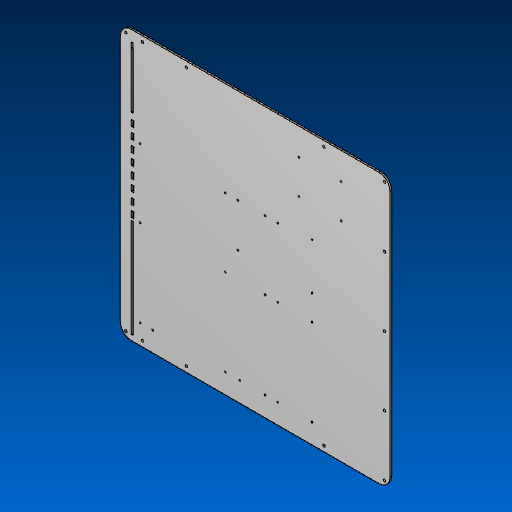
# Autodesk Inventor part: right_panel
Saved by Autodesk Inventor 2018 (Build 220112000, 112)
## iProperties
Created: 2019-10-14
Part Number: right_panel
Material: アルミニウム 6061
Document SubType Name: Modeling
Designer: gisen
Density: 2.7 g/cm^3
Appearance: アルミニウム - フラット
Author: gisen
Autodesk Inventor part; units mm, degrees
ref_plane "YZ Plane" through (0, 0, 0) normal (1, 0, 0) x (0, 1, 0)
ref_plane "XZ Plane" through (0, 0, 0) normal (0, 1, 0) x (-1, 0, 0)
ref_plane "XY Plane" through (0, 0, 0) normal (0, 0, 1) x (1, 0, 0)
sketch "スケッチ1" plane through (0, 0, 0) normal (0, 0, 1) x (1, 0, 0)
  line L0 (-225, -245) -> (225, -245)
  line L1 (245, -225) -> (245, 225)
  line L2 (225, 245) -> (-225, 245)
  line L3 (-245, 225) -> (-245, -225)
  line L4 (-245, -245) -> (245, 245) construction
  line L5 (245, -245) -> (-245, 245) construction
  circle A0 centre (-235, 235) radius 2.25
  circle A1 centre (235, 235) radius 2.25
  circle A2 centre (-235, -235) radius 2.25
  circle A3 centre (235, -235) radius 2.25
  arc A4 (-225, 245) -> (-245, 225) centre (-225, 225) ccw
  arc A5 (245, 225) -> (225, 245) centre (225, 225) ccw
  arc A6 (225, -245) -> (245, -225) centre (225, -225) ccw
  arc A7 (-245, -225) -> (-225, -245) centre (-225, -225) ccw
  point P0 (0, 0)
  dimension "d0" = 490
  dimension "d1" = 490
  dimension "d2" = 4.5
  dimension "d3" = 10
  dimension "d4" = 10
  dimension "d5" = 10
  dimension "d6" = 10
  dimension "d7" = 10
  dimension "d8" = 10
  dimension "d9" = 10
  dimension "d10" = 10
  dimension "d11" = 20
  constraints: 12 end point, 8 centre point, 8 point on circle, 8 point on line, 8 tangent, 6 equal radius, 2 midpoint, 2 parallel, 1 horizontal, 1 perpendicular
  measures "d0" distance of L5.end L4.end
  measures "d1" distance of L4.end L5.start
  measures "d2" diameter of A0
  measures "d3" distance from line of A0.centre L2
  measures "d4" distance from line of L3 A0.centre
  measures "d5" distance from line of A1.centre L2
  measures "d6" distance from line of L1 A1.centre
  measures "d7" distance from line of L1 A3.centre
  measures "d8" distance from line of L0 A3.centre
  measures "d9" distance from line of L0 A2.centre
  measures "d10" distance from line of L3 A2.centre
  measures "d11" radius of A4
extrude "押し出し1" add sketch "スケッチ1" along normal blind 3
sketch "スケッチ2" plane through (0, 0, 3) normal (0, 0, 1) x (1, 0, 0)
  circle A0 centre (18.0923, 72.9265) radius 1.6
  circle A1 centre (-54.2977, 72.9265) radius 1.6
  circle A2 centre (-209.2377, 72.9265) radius 1.6
  circle A3 centre (-209.2377, -51.5335) radius 1.6
  circle A4 centre (-186.3777, -209.0135) radius 1.6
  circle A5 centre (-54.2977, -209.0135) radius 1.6
  circle A6 centre (18.0923, -209.0135) radius 1.6
  circle A7 centre (18.0923, -51.5335) radius 1.6
  circle A8 centre (-54.2977, -51.5335) radius 1.6
  circle A9 centre (18.092, -209.014) radius 2.25 projected
  circle A10 centre (-186.378, -209.014) radius 2.25 projected
  circle A11 centre (18.092, -51.534) radius 2.25 projected
  circle A12 centre (18.092, 72.926) radius 2.25 projected
  circle A13 centre (-54.298, -209.014) radius 2.25 projected
  circle A14 centre (-54.298, -51.534) radius 2.25 projected
  circle A15 centre (-54.298, 72.926) radius 2.25 projected
  circle A16 centre (-209.238, -51.534) radius 2.25 projected
  circle A17 centre (-209.238, 72.926) radius 2.25 projected
  point P0 (0, 0)
  dimension "d14" = 3.2
  constraints: 9 centre point, 8 equal radius
  measures "d14" diameter of A0
extrude "押し出し2" cut sketch "スケッチ2" against normal blind 3 contours A0 | A1 | A2 | A3 | A4 | A5 | A6 | A7 | A8
sketch "スケッチ4" plane through (0, 0, 3) normal (0, 0, 1) x (1, 0, 0)
  line L0 (-225, -225) -> (-222, -225) projected
  line L1 (-225, -50.8937) -> (-225, -40.6067) projected
  line L2 (-225, -50.8937) -> (-222, -50.8937) projected
  line L3 (-222, -40.6067) -> (-222, -50.8937) projected
  line L4 (-225, -40.6067) -> (-222, -40.6067) projected
  line L5 (-225, -30.5483) -> (-225, -20.2613) projected
  line L6 (-225, -30.5483) -> (-222, -30.5483) projected
  line L7 (-222, -20.2613) -> (-222, -30.5483) projected
  line L8 (-225, -20.2613) -> (-222, -20.2613) projected
  line L9 (-225, -9.8937) -> (-225, 0.3933) projected
  line L10 (-225, -9.8937) -> (-222, -9.8937) projected
  line L11 (-222, 0.3933) -> (-222, -9.8937) projected
  line L12 (-225, 0.3933) -> (-222, 0.3933) projected
  line L13 (-225, 10.4517) -> (-225, 20.7387) projected
  line L14 (-225, 10.4517) -> (-222, 10.4517) projected
  line L15 (-222, 20.7387) -> (-222, 10.4517) projected
  line L16 (-225, 20.7387) -> (-222, 20.7387) projected
  line L17 (-225, 31.1063) -> (-225, 41.3933) projected
  line L18 (-225, 31.1063) -> (-222, 31.1063) projected
  line L19 (-222, 41.3933) -> (-222, 31.1063) projected
  line L20 (-225, 41.3933) -> (-222, 41.3933) projected
  line L21 (-225, 51.4517) -> (-225, 61.7387) projected
  line L22 (-225, 51.4517) -> (-222, 51.4517) projected
  line L23 (-222, 61.7387) -> (-222, 51.4517) projected
  line L24 (-225, 61.7387) -> (-222, 61.7387) projected
  line L25 (-225, 72.1063) -> (-225, 82.3933) projected
  line L26 (-225, 72.1063) -> (-222, 72.1063) projected
  line L27 (-222, 82.3933) -> (-222, 72.1063) projected
  line L28 (-225, 82.3933) -> (-222, 82.3933) projected
  line L29 (-225, 92.4517) -> (-225, 102.7387) projected
  line L30 (-225, 92.4517) -> (-222, 92.4517) projected
  line L31 (-222, 102.7387) -> (-222, 92.4517) projected
  line L32 (-225, 102.7387) -> (-222, 102.7387) projected
  line L33 (-225, 225) -> (-225, 132.6) projected
  line L34 (-225, 132.6) -> (-222, 132.6) projected
  line L35 (-222, 225) -> (-222, 132.6) projected
  line L36 (-225, 225) -> (-222, 225) projected
  line L37 (-222, 102.7387) -> (-221, 102.7387)
  line L38 (-221, 102.7387) -> (-221, 92.4517)
  line L39 (-221, 92.4517) -> (-222, 92.4517)
  line L40 (-222, 82.3933) -> (-221, 82.3933)
  line L41 (-221, 82.3933) -> (-221, 72.1063)
  line L42 (-221, 72.1063) -> (-222, 72.1063)
  line L43 (-222, 61.7387) -> (-221, 61.7387)
  line L44 (-221, 61.7387) -> (-221, 51.4517)
  line L45 (-221, 51.4517) -> (-222, 51.4517)
  line L46 (-222, 41.3933) -> (-221, 41.3933)
  line L47 (-221, 41.3933) -> (-221, 31.1063)
  line L48 (-221, 31.1063) -> (-222, 31.1063)
  line L49 (-222, 20.7387) -> (-221, 20.7387)
  line L50 (-221, 20.7387) -> (-221, 10.4517)
  line L51 (-221, 10.4517) -> (-222, 10.4517)
  line L52 (-222, 0.3933) -> (-221, 0.3933)
  line L53 (-221, 0.3933) -> (-221, -9.8937)
  line L54 (-221, -9.8937) -> (-222, -9.8937)
  line L55 (-222, -20.2613) -> (-221, -20.2613)
  line L56 (-221, -20.2613) -> (-221, -30.5483)
  line L57 (-221, -30.5483) -> (-222, -30.5483)
  line L58 (-222, -40.6067) -> (-221, -40.6067)
  line L59 (-221, -40.6067) -> (-221, -50.8937)
  line L60 (-221, -50.8937) -> (-222, -50.8937)
  line L61 (-225, -225) -> (-225, -56.064) projected
  line L62 (-222, -56.064) -> (-222, -225) projected
  line L63 (-225, -56.064) -> (-222, -56.064) projected
  point P0 (0, 0)
  point P1 (-225, -58.3552)
  point P2 (-222, -58.3552)
  point P3 (-225, -120.4005)
  point P4 (-222, -120.4005)
  dimension "d17" = 1
  constraints: 48 end point, 15 perpendicular, 8 horizontal, 7 parallel, 1 collinear, 2 other
  measures "d17" distance of L31.start L37.end
extrude "押し出し3" cut sketch "スケッチ4" against normal blind 3
sketch "スケッチ5" plane through (0, 0, 3) normal (0, 0, 1) x (1, 0, 0)
  circle A0 centre (-235, 235) radius 2.25 construction
  circle A1 centre (-235, -235) radius 2.25 construction
  circle A2 centre (-205, -235) radius 2.25
  line L0 (-225, -245) -> (225, -245) projected
  circle A3 centre (-205, 235) radius 2.25
  line L1 (225, 245) -> (-225, 245) projected
  point P0 (0, 0)
  dimension "d20" = 30
  dimension "d21" = 10
  dimension "d22" = 30
  dimension "d23" = 10
  constraints: 2 centre point, 2 equal radius
  measures "d20" distance of A1.centre A2.centre
  measures "d21" distance from line of L0 A2.centre
  measures "d22" distance of A0.centre A3.centre
  measures "d23" distance from line of L1 A3.centre
extrude "押し出し4" cut sketch "スケッチ5" against normal blind 3
sketch "スケッチ6" plane through (0, 0, 3) normal (0, 0, 1) x (1, 0, 0)
  circle A0 centre (-205, -235) radius 2.25 construction
  circle A1 centre (-205, 235) radius 2.25 construction
  circle A2 centre (18.0923, -51.5335) radius 1.6 construction
  circle A3 centre (-54.2977, -209.0135) radius 1.6 construction
  circle A4 centre (-209.2377, -51.5335) radius 1.6 construction
  circle A5 centre (-54.2977, 72.9265) radius 1.6 construction
  circle A6 centre (18.0923, 72.9265) radius 1.6 construction
  circle A7 centre (-209.2377, 72.9265) radius 1.6 construction
  circle A8 centre (-186.3777, -209.0135) radius 1.6 construction
  circle A9 centre (18.0923, -209.0135) radius 1.6 construction
  circle A10 centre (-54.2977, -51.5335) radius 1.6 construction
  circle A11 centre (235, -235) radius 2.25 construction
  circle A12 centre (-235, -235) radius 2.25 construction
  circle A13 centre (235, 235) radius 2.25 construction
  circle A14 centre (-235, 235) radius 2.25 construction
  line L0 (225, 245) -> (-225, 245) construction
  arc A15 (-225, 245) -> (-245, 225) centre (-225, 225) ccw construction
  line L1 (-245, 225) -> (-245, -225) construction
  arc A16 (-245, -225) -> (-225, -245) centre (-225, -225) ccw construction
  line L2 (-225, -245) -> (225, -245) construction
  arc A17 (225, -245) -> (245, -225) centre (225, -225) ccw construction
  line L3 (245, -225) -> (245, 225) construction
  arc A18 (245, 225) -> (225, 245) centre (225, 225) ccw construction
  line L4 (-221.75, 114.35) -> (-225.25, 114.35)
  line L5 (-225.25, 114.35) -> (-225.25, 215.25)
  line L6 (-225.25, 215.25) -> (-221.75, 215.25)
  line L7 (-221.75, 215.25) -> (-221.75, 114.35)
  line L8 (-220.75, 102.9892) -> (-220.75, 92.2022)
  line L9 (-220.75, 92.2022) -> (-225.25, 92.2022)
  line L10 (-225.25, 92.2022) -> (-225.25, 102.9892)
  line L11 (-225.25, 102.9892) -> (-220.75, 102.9892)
  line L12 (-220.75, 82.6438) -> (-220.75, 71.8568)
  line L13 (-220.75, 71.8568) -> (-225.25, 71.8568)
  line L14 (-225.25, 71.8568) -> (-225.25, 82.6438)
  line L15 (-225.25, 82.6438) -> (-220.75, 82.6438)
  line L16 (-220.75, 61.9892) -> (-220.75, 51.2022)
  line L17 (-220.75, 51.2022) -> (-225.25, 51.2022)
  line L18 (-225.25, 51.2022) -> (-225.25, 61.9892)
  line L19 (-225.25, 61.9892) -> (-220.75, 61.9892)
  line L20 (-220.75, 41.6438) -> (-220.75, 30.8568)
  line L21 (-220.75, 30.8568) -> (-225.25, 30.8568)
  line L22 (-225.25, 30.8568) -> (-225.25, 41.6438)
  line L23 (-225.25, 41.6438) -> (-220.75, 41.6438)
  line L24 (-220.75, 20.9892) -> (-220.75, 10.2022)
  line L25 (-220.75, 10.2022) -> (-225.25, 10.2022)
  line L26 (-225.25, 10.2022) -> (-225.25, 20.9892)
  line L27 (-225.25, 20.9892) -> (-220.75, 20.9892)
  line L28 (-220.75, 0.6438) -> (-220.75, -10.1432)
  line L29 (-220.75, -10.1432) -> (-225.25, -10.1432)
  line L30 (-225.25, -10.1432) -> (-225.25, 0.6438)
  line L31 (-225.25, 0.6438) -> (-220.75, 0.6438)
  line L32 (-220.75, -20.0108) -> (-220.75, -30.7978)
  line L33 (-220.75, -30.7978) -> (-225.25, -30.7978)
  line L34 (-225.25, -30.7978) -> (-225.25, -20.0108)
  line L35 (-225.25, -20.0108) -> (-220.75, -20.0108)
  line L36 (-220.75, -40.3562) -> (-220.75, -51.1432)
  line L37 (-220.75, -51.1432) -> (-225.25, -51.1432)
  line L38 (-225.25, -51.1432) -> (-225.25, -40.3562)
  line L39 (-225.25, -40.3562) -> (-220.75, -40.3562)
  line L40 (-221.75, -55.8135) -> (-225.25, -55.8135)
  line L41 (-225.25, -55.8135) -> (-225.25, -235.25)
  line L42 (-225.25, -235.25) -> (-221.75, -235.25)
  line L43 (-221.75, -235.25) -> (-221.75, -55.8135)
  line L44 (-225, -30.5483) -> (-225, -20.2613) projected
  line L45 (-222, -56.064) -> (-222, -225) projected
  line L46 (-225, 0.3933) -> (-221, 0.3933) projected
  line L47 (-221, 0.3933) -> (-221, -9.8937) projected
  line L48 (-221, -9.8937) -> (-225, -9.8937) projected
  line L49 (-225, 102.7387) -> (-221, 102.7387) projected
  line L50 (-221, 102.7387) -> (-221, 92.4517) projected
  line L51 (-221, 92.4517) -> (-225, 92.4517) projected
  line L52 (-225, 82.3933) -> (-221, 82.3933) projected
  line L53 (-221, 82.3933) -> (-221, 72.1063) projected
  line L54 (-221, 72.1063) -> (-225, 72.1063) projected
  line L55 (-225, 61.7387) -> (-221, 61.7387) projected
  line L56 (-221, 61.7387) -> (-221, 51.4517) projected
  line L57 (-221, 51.4517) -> (-225, 51.4517) projected
  line L58 (-225, 41.3933) -> (-221, 41.3933) projected
  line L59 (-221, 41.3933) -> (-221, 31.1063) projected
  line L60 (-221, 31.1063) -> (-225, 31.1063) projected
  line L61 (-225, 20.7387) -> (-221, 20.7387) projected
  line L62 (-221, 20.7387) -> (-221, 10.4517) projected
  line L63 (-221, 10.4517) -> (-225, 10.4517) projected
  line L64 (-225, 225) -> (-222, 225) projected
  line L65 (-225, 92.4517) -> (-225, 102.7387) projected
  line L66 (-225, 51.4517) -> (-225, 61.7387) projected
  line L67 (-225, 10.4517) -> (-225, 20.7387) projected
  line L68 (-225, 31.1063) -> (-225, 41.3933) projected
  line L69 (-225, 72.1063) -> (-225, 82.3933) projected
  line L70 (-222, 132.6) -> (-225, 132.6) projected
  line L71 (-225, 132.6) -> (-225, 225) projected
  line L72 (-222, -225) -> (-225, -225) projected
  line L73 (-225, -225) -> (-225, -56.064) projected
  line L74 (-225, -56.064) -> (-222, -56.064) projected
  line L75 (-222, 225) -> (-222, 132.6) projected
  line L76 (-225, -9.8937) -> (-225, 0.3933) projected
  line L77 (-221, -30.5483) -> (-225, -30.5483) projected
  line L78 (-225, -20.2613) -> (-221, -20.2613) projected
  line L79 (-221, -20.2613) -> (-221, -30.5483) projected
  point P0 (0, 0)
  constraints: 80 end point
extrude "押し出し5" cut sketch "スケッチ6" against normal through all contours L4 L5 L6 L71 L70 L75 L7 | L75 L70 L71 L6 | L8 L9 L10 L11 | L12 L13 L14 L15 | L16 L17 L18 L19 | L20 L21 L22 L23 | L24 L25 L26 L27 | L28 L29 L30 L31 | L32 L33 L34 L35 | L36 L37 L38 L39 | L43 L42 L41 L40 | L44 L78 L79 L77 | L45 L72 L73 L74 | L46 L47 L48 L76 | L49 L50 L51 L65 | L52 L53 L54 L69 | L55 L56 L57 L66 | L58 L59 L60 L68 | L61 L62 L63 L67
sketch "スケッチ7" plane through (0, 0, 3) normal (0, 0, 1) x (1, 0, 0)
  line L0 (245, 225) -> (245, -225) projected
  circle A0 centre (-125, -235) radius 2.25 projected
  circle A1 centre (235, 0) radius 2.25 projected
  circle A2 centre (125, -235) radius 2.25 projected
  circle A3 centre (235, 125) radius 2.25 projected
  circle A4 centre (-125, 235) radius 2.25 projected
  circle A5 centre (-235, -125) radius 2.25 projected
  circle A6 centre (-235, 0) radius 2.25 projected
  circle A7 centre (125, 235) radius 2.25 projected
  circle A8 centre (235, -125) radius 2.25 projected
  line L1 (-225.2, 124.9816) -> (-221.8, 124.9816) projected
  line L2 (-221.8, 124.9816) -> (-221.8, 225.2) projected
  line L3 (-221.8, 225.2) -> (-225.2, 225.2) projected
  line L4 (-225.2, 225.2) -> (-225.2, 124.9816) projected
  circle A9 centre (-235, 125) radius 2.25 projected
  circle A10 centre (235, 235) radius 2.25 projected
  circle A11 centre (-235, 235) radius 2.25 projected
  circle A12 centre (235, -235) radius 2.25 projected
  circle A13 centre (-235, -235) radius 2.25 projected
  line L5 (225, -245) -> (-225, -245) projected
  arc A14 (-245, -225) -> (-225, -245) centre (-225, -225) ccw projected
  line L6 (-245, -225) -> (-245, 225) projected
  arc A15 (-225, 245) -> (-245, 225) centre (-225, 225) ccw projected
  line L7 (-225, 245) -> (225, 245) projected
  arc A16 (245, 225) -> (225, 245) centre (225, 225) ccw projected
  line L8 (245, 225) -> (245, -225) projected
  arc A17 (225, -245) -> (245, -225) centre (225, -225) ccw projected
  point P0 (0, 0)
extrude "押し出し6" cut sketch "スケッチ7" against normal up to surface (3 mm away) contours A0 | A1 | A2 | A3 | A4 | A7 | A8
sketch "スケッチ8" plane through (0, 0, 0) normal (0, 0, -1) x (-1, 0, 0)
  line L0 (-69.775, 130.075) -> (-170.225, 130.075) construction
  line L1 (-170.225, 130.075) -> (-170.225, 199.925) construction
  line L2 (-170.225, 199.925) -> (-69.775, 199.925) construction
  line L3 (-69.775, 199.925) -> (-69.775, 130.075) construction
  line L4 (-69.775, 130.075) -> (-170.225, 199.925) construction
  line L5 (-170.225, 130.075) -> (-69.775, 199.925) construction
  line L6 (225, 245) -> (-225, 245) construction
  line L7 (-245, 225) -> (-245, -225) construction
  line L8 (-79.625, 195.86) -> (-156.225, 195.86) construction
  line L9 (-156.225, 195.86) -> (-156.225, 134.14) construction
  line L10 (-156.225, 134.14) -> (-79.625, 134.14) construction
  line L11 (-79.625, 134.14) -> (-79.625, 195.86) construction
  line L12 (-79.625, 195.86) -> (-156.225, 134.14) construction
  line L13 (-156.225, 195.86) -> (-79.625, 134.14) construction
  line L14 (-117.925, 165) -> (-120, 165) construction
  circle A0 centre (-79.625, 134.14) radius 1.6
  circle A1 centre (-79.625, 195.86) radius 1.6
  circle A2 centre (-156.225, 195.86) radius 1.6
  circle A3 centre (-156.225, 134.14) radius 1.6
  point P0 (0, 0)
  dimension "d40" = 69.85
  dimension "d41" = 100.45
  dimension "d42" = 80
  dimension "d43" = 125
  dimension "d44" = 61.72
  dimension "d45" = 90.6
  dimension "d46" = 14
  dimension "d47" = 3.2
  dimension "d48" = 3.2
  dimension "d49" = 3.2
  dimension "d50" = 3.2
  constraints: 26 end point, 4 centre point, 4 coincident, 4 midpoint, 4 parallel, 3 horizontal, 2 perpendicular
  measures "d40" distance of L0.end L1.end
  measures "d41" distance of L0.start L0.end
  measures "d42" distance from line of L6 L14.end
  measures "d43" distance from line of L7 L14.end
  measures "d44" distance of L10.end L8.start
  measures "d45" distance between parallel lines of L1 L11
  measures "d46" distance between parallel lines of L1 L9
  measures "d47" diameter of A0
  measures "d48" diameter of A1
  measures "d49" diameter of A2
  measures "d50" diameter of A3
extrude "押し出し7" cut sketch "スケッチ8" against normal through all
sketch "スケッチ9" plane through (0, 0, 0) normal (0, 0, -1) x (-1, 0, 0)
  circle A0 centre (186.3777, -209.0135) radius 1.6 construction
  circle A1 centre (54.2977, -209.0135) radius 1.6 construction
  circle A2 centre (-18.0923, -209.0135) radius 1.6 construction
  circle A3 centre (209.2377, -51.5335) radius 1.6 construction
  circle A4 centre (209.2377, 72.9265) radius 1.6 construction
  circle A5 centre (54.2977, 72.9265) radius 1.6 construction
  circle A6 centre (-18.0923, 72.9265) radius 1.6 construction
  circle A7 centre (54.2977, -51.5335) radius 1.6 construction
  circle A8 centre (-18.0923, -51.5335) radius 1.6 construction
  line L0 (219.3977, -215.3635) -> (-52.3823, -215.3635) construction
  line L1 (-52.3823, -215.3635) -> (-52.3823, 89.4365) construction
  line L2 (-52.3823, 89.4365) -> (219.3977, 89.4365) construction
  line L3 (219.3977, 89.4365) -> (219.3977, -215.3635) construction
  point P0 (0, 0)
  dimension "d53" = 6.35
  dimension "d54" = 33.02
  dimension "d55" = 304.8
  dimension "d56" = 271.78
  constraints: 8 end point, 2 parallel, 1 horizontal, 1 perpendicular
  measures "d53" distance from line of A0.centre L0
  measures "d54" distance from line of L3 A0.centre
  measures "d55" distance of L2.end L0.start
  measures "d56" distance of L0.start L0.end
sketch "スケッチ10" plane through (0, 0, 0) normal (0, 0, -1) x (-1, 0, 0)
  line L0 (219.3977, -215.3635) -> (-110.8023, -215.3635) construction
  line L1 (-110.8023, -215.3635) -> (-110.8023, 89.4365) construction
  line L2 (-110.8023, 89.4365) -> (219.3977, 89.4365) construction
  line L3 (219.3977, 89.4365) -> (219.3977, -215.3635) construction
  circle A0 centre (209.2377, 72.9265) radius 1.6 construction
  circle A1 centre (-235, -125) radius 2.25 projected
  circle A2 centre (-103.1823, 78.0065) radius 1.6
  circle A3 centre (209.2377, 72.9265) radius 1.6 construction
  line L4 (209.2377, 72.9265) -> (54.2977, 72.9265) construction
  circle A4 centre (54.2977, 72.9265) radius 1.6 construction
  circle A5 centre (54.2977, 72.9265) radius 1.6 construction
  line L5 (54.2977, 72.9265) -> (-18.0923, 72.9265) construction
  line L6 (-18.0923, 72.9265) -> (-40.9523, 72.9265) construction
  circle A6 centre (-18.0923, 72.9265) radius 1.6
  circle A7 centre (-40.9523, 72.9265) radius 1.6
  line L7 (-103.1823, 78.0065) -> (-103.1823, -5.8135) construction
  line L8 (-103.1823, -5.8135) -> (-103.1823, -51.5335) construction
  line L9 (-103.1823, -51.5335) -> (-103.1823, -208.9135) construction
  circle A8 centre (-103.1823, -5.8135) radius 1.6
  circle A9 centre (-103.1823, -51.5335) radius 1.6
  circle A10 centre (-103.1823, -208.9135) radius 1.6
  line L10 (-103.1823, -5.8135) -> (31.4377, -5.8135) construction
  circle A11 centre (31.4377, -5.8135) radius 1.6
  line L11 (31.4377, -5.8135) -> (31.4377, 72.9265) construction
  circle A12 centre (31.4377, 72.9265) radius 1.6
  line L12 (209.2377, 72.9265) -> (209.2377, -209.0135) construction
  circle A13 centre (186.3777, -209.0135) radius 1.6 construction
  line L13 (209.2377, -209.0135) -> (186.3777, -209.0135) construction
  circle A14 centre (209.2377, -209.0135) radius 1.6
  line L14 (-40.9523, 72.9265) -> (-40.9523, -209.0135) construction
  line L15 (-40.9523, -209.0135) -> (-18.0923, -209.0135) construction
  circle A15 centre (-18.0923, -51.5335) radius 1.6 construction
  line L16 (-18.0923, -51.5335) -> (-40.9523, -51.5335) construction
  circle A16 centre (-18.0923, -209.0135) radius 1.6 construction
  circle A17 centre (-40.9523, -51.5335) radius 1.6
  circle A18 centre (-40.9523, -209.0135) radius 1.6
  line L17 (-18.0923, -209.0135) -> (186.3777, -209.0135) construction
  circle A19 centre (27.6277, -209.0135) radius 1.6
  point P0 (0, 0)
  dimension "d57" = 330.2
  dimension "d58" = 304.8
  dimension "d59" = 10.16
  dimension "d60" = 16.51
  dimension "d61" = 124.1977
  dimension "d62" = 5.08
  dimension "d63" = 312.42
  dimension "d64" = 154.94
  dimension "d65" = 227.33
  dimension "d66" = 250.19
  dimension "d67" = 78.74
  dimension "d68" = 124.46
  dimension "d69" = 281.84
  dimension "d70" = 177.8
  dimension "d71" = 134.62
  dimension "d72" = 16.51
  dimension "d73" = 181.61
  dimension "d74" = 3.2
  constraints: 36 end point, 14 centre point, 13 coincident, 13 equal radius, 6 point on line, 5 horizontal, 4 perpendicular, 4 vertical, 2 parallel
  measures "d57" distance of L0.start L0.end
  measures "d58" distance of L0.end L1.end
  measures "d59" distance from line of A0.centre L3
  measures "d60" distance from line of L2 A0.centre
  measures "d61" distance from line of L1 A1.centre
  measures "d62" vertical distance of A0.centre L7.start
  measures "d63" horizontal distance of A0.centre L7.start
  measures "d64" distance of L4.start L4.end
  measures "d65" distance of L5.end L4.start
  measures "d66" distance of L4.start L6.end
  measures "d67" vertical distance of L10.start A0.centre
  measures "d68" vertical distance of L8.end A0.centre
  measures "d69" vertical distance of L4.start L9.end
  measures "d70" horizontal distance of L4.start L10.end
  measures "d71" distance of L10.start L10.end
  measures "d72" distance from line of L2 L11.end
  measures "d73" distance from line of L12 A19.centre
  measures "d74" diameter of A0
extrude "押し出し8" cut sketch "スケッチ10" against normal blind 10 contours A2 | A7 | A8 | A9 | A10 | A11 | A12 | A14 | A17 | A18 | A19
equation "\"d5\" = d3"
equation "\"d6\" = d4"
equation "\"d7\" = d6"
equation "\"d8\" = d5"
equation "\"d9\" = d8"
equation "\"d10\" = d7"
